Autodesk Fusion 360 part; units mm, degrees
note: some values were not read from the file. Set by a fixed rule: which sketch regions a step uses.
(part 3 of 3)
  constraint equal A462 A463
  constraint coincident P17 L940
  constraint coincident P17 L941
  constraint tangent L940 A464
  constraint tangent L941 A464
  constraint equal A462 A464
  constraint coincident P16 L939
  constraint coincident P16 L940
  constraint tangent L939 A465
  constraint tangent L940 A465
  constraint equal A462 A465
  constraint tangent A79 L947
  constraint concentric A453 A466
  constraint tangent A455 A466
  constraint concentric A459 A469
  constraint concentric A460 A468
  constraint concentric A461 A467
  constraint concentric A454 A470
  constraint vertical L948
  constraint tangent A466 L949
  constraint vertical L949
  constraint perpendicular L944 L950
  constraint tangent L951 A468
  constraint coincident L953.start A470
  constraint tangent L953 A470
  constraint horizontal L953
  constraint concentric A470 A471
  constraint tangent L948 A472
  constraint tangent A469 A472
  constraint tangent L948 A473
  constraint tangent A468 A473
  constraint tangent L950 A474
  constraint tangent A467 A474
  constraint tangent L949 A475
  constraint tangent L950 A475
  constraint tangent L958 A483
  constraint perpendicular L941 L958
  constraint tangent L959 A483
  constraint perpendicular L941 L959
  constraint tangent L960 A485
  constraint tangent L961 A485
  constraint concentric A458 A490
  constraint tangent L952 A490
  constraint tangent A471 L966
  constraint vertical L966
  constraint perpendicular L966 L967
  constraint tangent L967 A491
  constraint tangent A490 A491
  constraint tangent L966 A492
  constraint tangent L967 A492
  measures "d35" radius of A2
  measures "d36" radius of A3
  measures "d40" distance of L16.start L16.end
  measures "d41" radius of A4
  measures "d67" radius of A23
  measures "d68" distance of L75.start L75.end
  measures "d69" radius of A27
  measures "d89" radius of A39
  measures "d94" radius of A40
  measures "d112" diameter of A42
  measures "d113" diameter of A43
  measures "d116" radius of A46
  measures "d369" radius of A64
  measures "d426" diameter of A86
  measures "d427" diameter of A87
  measures "d429" radius of A88
  measures "d466" radius of A94
  measures "d474" radius of A96
  measures "d508" radius of A98
  measures "d524" diameter of A105
  measures "d525" diameter of A104
  measures "d526" radius of A106
  measures "d527" radius of A108
  measures "d528" radius of A110
  measures "d529" radius of A112
  measures "d532" distance of L341.start L341.end
  measures "d533" distance of L341.start L343.end
  measures "d534" distance of L345.start L345.end
  measures "d535" distance of L345.start L347.end
  measures "d545" radius of A118
  measures "d546" radius of A120
  measures "d555" radius of A132
  measures "d557" radius of A141
  measures "d575" radius of A145
  measures "d576" radius of A146
  measures "d577" radius of A147
  measures "d578" radius of A148
  measures "d579" radius of A177
  measures "d589" distance of L568.start L568.end
  measures "d591" radius of A178
  measures "d592" radius of A179
  measures "d593" radius of A180
  measures "d594" radius of A181
  measures "d604" radius of A190
  measures "d605" radius of A191
  measures "d625" diameter of A194
  measures "d629" radius of A197
  measures "d643" radius of A201
  measures "d648" radius of A209
  measures "d649" radius of A211
  measures "d652" radius of A224
  measures "d654" radius of A243
  measures "d655" radius of A244
  measures "d675" radius of A247
  measures "d686" radius of A249
  measures "d687" radius of A251
  measures "d688" distance of L685.start L722.end
  measures "d693" diameter of A292
  measures "d694" diameter of A293
  measures "d695" diameter of A294
  measures "d701" diameter of A295
  measures "d703" diameter of A297
  measures "d704" diameter of A298
  measures "d705" diameter of A299
  measures "d706" diameter of A300
  measures "d707" diameter of A301
  measures "d709" radius of A302
  measures "d718" diameter of A317
  measures "d719" diameter of A318
  measures "d722" radius of A319
  measures "d726" diameter of A327
  measures "d727" diameter of A328
  measures "d728" diameter of A329
  measures "d729" radius of A330
  measures "d742" radius of A375
  measures "d750" radius of A396
  measures "d772" diameter of A411
  measures "d773" radius of A413
  measures "d774" radius of A423
  measures "d861" diameter of A436
  measures "d862" diameter of A437
  measures "d863" diameter of A438
  measures "d864" diameter of A439
  measures "d865" radius of A444
  measures "d872" diameter of A452
  measures "d873" diameter of A453
  measures "d876" diameter of A454
  measures "d882" radius of A455
  measures "d899" distance of L938.start P15
  measures "d901" distance of P16 P17
  measures "d902" radius of A462
  measures "d910" diameter of A469
  measures "d912" diameter of A468
  measures "d913" diameter of A467
  measures "d914" diameter of A470
  measures "d916" radius of A474
  measures "d918" radius of A475
  measures "d921" diameter of A482
  measures "d922" diameter of A483
  measures "d923" diameter of A484
  measures "d924" diameter of A485
  measures "d925" radius of A491
  measures "d926" radius of A492
extrude "Estrusione12" add sketch "Schizzo1" along normal blind 5 contours L4 L5 L6 L7 A0 A1 A3 L16 L17 L18 L19 A4 A5 A6 L24 A7 L25 L26 L27 L28 A8 L29 A9 L30 A10 L31 A11 L40 A12 L41 A13 L42 A14 L43 A15 L44 L45 L54 L55 L56 L57 L58 L59 A16 L60 A17 L61 A18 L62 A19 L63 A20 L563 L564 L844 L845 L846 L847 L848 L849 | L8 L9 A2 L10 L11 L12 L13 L14 L15 L80 A31 L81 L82 L83 L84 L85 L86 L87 L88 L89 A32 L90 L91 A33 L98 L99 L100 L349 L350 L594 L595 A184 L596 A185 L600 L601 A186 L602 A187 L603 L604 L605 L606 L607 L608 | L72 L73 L75 A21 A22 A23 A24 A25 L76 L77 A26 A27 L78 L79 A28 A29 A30 L142 L143 L144 L351 L352 L353 A114 A115 A116 A117 L354 L355 L356 L357 L358 A118 A119 A120 A121 L359 A122 L360 A123 L361 A124 A125 L362 L363 A126 A127 L364 A128 A129 L365 L565 L814 A341 L815 A342 L816 A343 A344 L817 A345 A346 L818 A347 L819 A348 L820 A349 L821 A350 L822 A351 L823 A352 L824 A353 L825 L826 A354 L827 A355 L828 A356 L829 A357 L830 A358 L831 A359 L832 A360 L833 A361 A362 L834 A363 A364 L835 A365 L836 A366 L837 L838 L839 L896 L897 L898 A423 A424 L902 A429 L907 L908 A430 L909 L910 L911 A431 A432 L914 L915 L918 L920 L921 L924 L925 L928 | L101 L102 L103 L105 L106 L107 L108 L109 L110 L111 A34 L112 L113 L114 L115 L116 L117 L118 L121 A35 A36 A37 L123 L124 L125 L126 L127 L128 L129 L130 L131 A38 L133 L134 L135 L136 A39 A40 A41 L333 L334 L584 L585 L586 A182 L588 A183 L589 L592 | L307 L308 L309 L310 L311 A79 L312 L313 L314 L316 L317 L318 L319 L320 L321 L566 L567 L754 L755 L778 L779 L780 L781 L782 L783 L784 L785 L786 L787 L788 L789 L790 A314 A315 L791 L792 L793 L794 A316 L795 L796 A412 A413 A414 A415 A416 A417 A419 A420 L947 | L577 L578 L580 L581 A178 A179 A180 A181 A240 A241 A242 A243 A244 A246 A247 A248 | L645 L646 L647 L648 L649 A190 A191 A192 A193 A201 | L766 A310 L769 makes body 1 at (-95.6667, 0, -8.3333) makes body 2 at (-442.5613, 0, -103.6472) makes body 3 at (-83.3644, 0, 38.8224) makes body 4 at (33.2673, 0, -128.6547) makes body 5 at (-219.7749, 0, -101.6667) makes body 6 at (5, 0, 54.7069) makes body 7 at (26.6667, 0, 43.6243)
extrude "Extrude20" add sketch "Schizzo1" along normal blind 2 separate body contours A454 L934 L935 A455 A456 A457 A466 L948 L949 L950 L951 L952 A467 A468 A469 L953 A470 A471 A472 A473 A474 A475 L966 L967 A490 A491 A492 A493 L968 A494 A495 L969 A496 L970 A497 A498 L971 A499 A500 L972 A501 A502 L973 A503 A504 L974 A505 L975 A506 L976 A507 A508 L977 makes body 8
